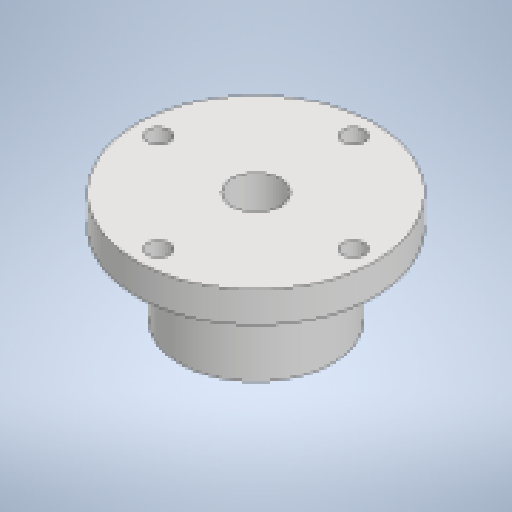
# Autodesk Inventor part: 8 mm hub
Saved by Autodesk Inventor 2025 (Build 290162000, 162)
## iProperties
Created: 2025-07-04
Part Number: 8 mm hub
Material: 一般
Document SubType Name: Modeling
Designer: gavin
Density: 1 g/cm^3
Appearance: 預設
Author: gavin
Autodesk Inventor part; units mm, degrees
ref_plane "YZ Plane" through (0, 0, 0) normal (1, 0, 0) x (0, 1, 0)
ref_plane "XZ Plane" through (0, 0, 0) normal (0, 1, 0) x (-1, 0, 0)
ref_plane "XY Plane" through (0, 0, 0) normal (0, 0, 1) x (1, 0, 0)
sketch "草圖1" plane through (0, 0, 0) normal (0, 1, 0) x (-1, 0, 0)
  circle A0 centre (0, 0) radius 4
  circle A1 centre (0, 0) radius 12.5
  dimension "d0" = 8
  dimension "d1" = 25
  constraints: 2 centre point, 2 coincident
  measures "d0" diameter of A0
  measures "d1" diameter of A1
extrude "擠出1" add sketch "草圖1" along normal blind 13
sketch "草圖2" plane through (0, 13, 0) normal (0, 1, 0) x (1, 0, 0)
  circle A0 centre (0, 0) radius 19.5
  circle A1 centre (0, 0) radius 4 projected
  dimension "d4" = 39
  constraints: 1 centre point, 1 coincident
  measures "d4" diameter of A0
extrude "擠出2" add sketch "草圖2" along normal blind 5
sketch "草圖3" plane through (0, 18, 0) normal (0, 1, 0) x (1, 0, 0)
  circle A0 centre (0, 0) radius 16 construction
  circle A1 centre (-16, 0) radius 1.75
  circle A2 centre (0, -16) radius 1.75
  circle A3 centre (16, 0) radius 1.75
  circle A4 centre (0, 16) radius 1.75
  dimension "d7" = 32
  dimension "d8" = 3.5
  dimension "d11" = 360
  constraints: 4 centre point, 1 coincident, 1 horizontal alignment, 11 other
  measures "d8" diameter of A1
extrude "擠出3" cut sketch "草圖3" against normal blind 5
